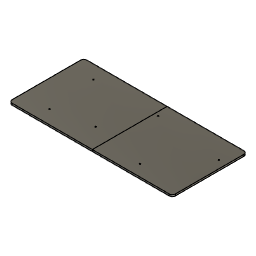
Rectangle DIY Case Backplate (Autodesk Fusion 360 design; units mm, degrees)
Autodesk Fusion 360 part; units mm, degrees
sketch "Sketch2" plane through (0, 0, -17.8) normal (0, 0, -1) x (1, 0, 0)
  arc A0 (-203.75, 114.9854) -> (-210.8339, 108) centre (-203.8478, 108) ccw
  line L0 (-210.8339, 108) -> (-210.8339, -42)
  arc A1 (-210.8339, -42) -> (-203.75, -48.9532) centre (-203.75, -41.8681) ccw
  line L1 (-203.75, -48.9532) -> (140, -48.9532)
  arc A2 (140, -48.9532) -> (146.9841, -42) centre (140.0308, -42) ccw
  line L2 (146.9841, -42) -> (146.9841, 108)
  arc A3 (146.9841, 108) -> (140, 114.9854) centre (140, 108.0013) ccw
  line L3 (140, 114.9854) -> (-203.75, 114.9854)
  arc A4 (-210.7339, -41.9991) -> (-203.75, -48.8532) centre (-203.75, -41.8681) ccw
  line L4 (-203.75, -48.8532) -> (140.0002, -48.8532)
  arc A5 (140.0002, -48.8532) -> (146.8841, -42) centre (140.0308, -42) ccw
  line L5 (146.8841, -42) -> (146.8841, 108)
  arc A6 (146.8841, 108) -> (140, 114.8854) centre (140, 108.0013) ccw
  line L6 (140, 114.8854) -> (-203.7507, 114.8854)
  arc A7 (-203.7507, 114.8854) -> (-210.7339, 108) centre (-203.8478, 108) ccw
  line L7 (-210.7339, 108) -> (-210.7339, -41.9991)
  circle A8 centre (-20, -21) radius 4
  circle A9 through (134, -4, 2.171) (128, -0.5359, 2.171) (128, -7.4641, 2.171)
  circle A10 through (-148, 85, -3.129) (-154, 88.4641, -3.129) (-154, 81.5359, -3.129)
  circle A11 through (-64, 68, -3.129) (-70, 71.4641, -3.129) (-70, 64.5359, -3.129)
  circle A12 through (55, 90, -3.129) (49, 93.4641, -3.129) (49, 86.5359, -3.129)
  circle A13 through (-16, -21, -3.129) (-22, -17.5359, -3.129) (-22, -24.4641, -3.129)
  circle A14 centre (130, -4) radius 4
  point P0 (-160, -19)
  dimension "d2" = -0.1
  dimension "d5" = 8
  dimension "d6" = 8
  dimension "d7" = 8
  dimension "d8" = 8
  dimension "d9" = 8
  dimension "d10" = 8
  dimension "d12" = 8
  measures "d5" diameter of A8
  measures "d12" diameter of A14
extrude "Extrude1" add sketch "Sketch2" along normal blind 2.2 contours A4 L4 A5 L5 A6 L6 A7 L7 | A8 | A14 makes body 1
sketch "Sketch4" plane through (0, 0, -20) normal (0, 0, -1) x (1, 0, 0)
  circle A0 centre (-160, -19) radius 4
  circle A1 centre (-68, 68) radius 4
  circle A2 centre (51, 90) radius 4
  circle A3 centre (-152, 85) radius 4
  line L0 (-210.7339, 108) -> (-210.7339, -41.9991)
  arc A4 (-210.7339, -41.9991) -> (-203.75, -48.8532) centre (-203.75, -41.8681) ccw
  line L1 (-203.75, -48.8532) -> (140.0002, -48.8532)
  arc A5 (140.0002, -48.8532) -> (146.8841, -42) centre (140.0308, -42) ccw
  line L2 (146.8841, -42) -> (146.8841, 108)
  arc A6 (146.8841, 108) -> (140, 114.8854) centre (140, 108.0013) ccw
  line L3 (140, 114.8854) -> (-203.7507, 114.8854)
  arc A7 (-203.7507, 114.8854) -> (-210.7339, 108) centre (-203.8478, 108) ccw
  circle A8 centre (-20, -21) radius 4
  circle A9 centre (130, -4) radius 4
  dimension "d11" = 8
  dimension "d13" = 8
  dimension "d14" = 8
  dimension "d15" = 8
  dimension "d16" = 8
  dimension "d17" = 8
  measures "d11" diameter of A0
  measures "d13" diameter of A1
  measures "d14" diameter of A2
  measures "d15" diameter of A3
  measures "d16" diameter of A8
  measures "d17" diameter of A9
hole "Hole1" at (-152, -85, -20) at (-68, -68, -20) at (-160, 19, -20) at (-20, 21, -20) at (51, -90, -20) at (130, 4, -20) direction (0, 0, 1) diameter 2.7 depth 36.85 tip angle 118 countersink diameter 8 countersink angle 120 bodies 1
extrude "Extrude2" add 1 faces at (53.6667, -21.3448, -17.8) along direction (0, 0, 1) blind 1.5 on bodies 1 bodies 1
extrude "Extrude3" cut 1 faces at (53.6667, -21.3448, -16.3) along direction (0, 0, -1) blind 0.7 on bodies 1 bodies 1
sketch "Sketch6" plane through (0, 0, -17) normal (0, 0, 1) x (-1, 0, 0)
  line L0 (28.2401, -50.0149) -> (28.2401, 114.9851)
  constraint vertical L0
sketch "Sketch7" plane through (0, 0, -17) normal (0, 0, 1) x (-1, 0, 0)
  circle A0 centre (-51, 90) radius 1.35
  circle A1 centre (160, -19) radius 1.35
  circle A2 centre (152, 85) radius 1.35
  circle A3 centre (68, 68) radius 1.35
  circle A4 centre (20, -21) radius 1.35
  circle A5 centre (-130, -4) radius 1.35
  line L0 (210.7339, -41.9991) -> (210.7339, 108)
  arc A6 (210.7339, 108) -> (203.7507, 114.8854) centre (203.8478, 108) ccw
  line L1 (203.7507, 114.8854) -> (-140, 114.8854)
  arc A7 (-140, 114.8854) -> (-146.8841, 108) centre (-140, 108.0013) ccw
  line L2 (-146.8841, 108) -> (-146.8841, -42)
  arc A8 (-146.8841, -42) -> (-140.0002, -48.8532) centre (-140.0308, -42) ccw
  line L3 (-140.0002, -48.8532) -> (203.75, -48.8532)
  arc A9 (203.75, -48.8532) -> (210.7339, -41.9991) centre (203.75, -41.8681) ccw
  line L4 (31.8749, -48.8532) -> (223.5444, -48.8532)
  line L5 (223.5444, -48.8532) -> (223.5444, 130.8995)
  line L6 (223.5444, 130.8995) -> (31.8749, 130.8995)
  line L7 (31.8749, 130.8995) -> (31.8749, -48.8532)
  line L8 (31.8749, -48.8532) -> (-156.0679, -48.8532)
  line L9 (-156.0679, -48.8532) -> (-156.0679, 130.2955)
  line L10 (-156.0679, 130.2955) -> (31.8749, 130.2955)
  line L11 (31.8749, 130.2955) -> (31.8749, -48.8532)
  constraint horizontal L4
  constraint vertical L5
  constraint horizontal L6
  constraint vertical L7
  constraint midpoint L3 L4.start
  constraint horizontal L8
  constraint vertical L9
  constraint horizontal L10
  constraint vertical L11
split "Split2" by curves path "Sketch7" along L5 L6 L7 L4 bodies 1 makes body 2 at (53.6132, -21.5198, -17)
extrude "Extrude4" add 2 faces at (-86.3357, 0.2958, -17) (53.6132, -21.5198, -17) along direction (0, 0, 1) blind 0.7 on bodies 1 2 bodies 1 2
split "Split3" by curves path "Sketch6" along L0 bodies 1 makes body 3 at (-85.1241, 0.2958, -16.3)
